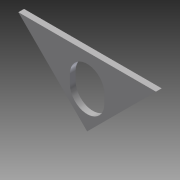
# Autodesk Inventor part: GE-13020-02
Saved by Autodesk Inventor 2013 (Build 170138000, 138)
## iProperties
Created: 2013-01-06
Part Number: GE-13020-02
Material: Steel
Document SubType Name: Modeling
Designer: Phillip
Density: 1 g/cm^3
Author: Phillip
Autodesk Inventor part; units mm, degrees
ref_plane "YZ Plane" through (0, 0, 0) normal (1, 0, 0) x (0, 1, 0)
ref_plane "XZ Plane" through (0, 0, 0) normal (0, 1, 0) x (-1, 0, 0)
ref_plane "XY Plane" through (0, 0, 0) normal (0, 0, 1) x (1, 0, 0)
sketch "Sketch1" plane through (0, 0, 0) normal (0, 0, 1) x (1, 0, 0)
  line L0 (0, 0) -> (-76.2, 76.2)
  line L1 (-76.2, 76.2) -> (76.2, 76.2)
  line L2 (76.2, 76.2) -> (0, 0)
  point P0 (0, 76.2)
  dimension "d0" = 152.4
  dimension "d2" = 76.2
  constraints: 6 end point, 1 horizontal, 1 midpoint, 1 vertical alignment
  measures "d0" distance of L0.end L1.end
  measures "d2" distance from line of L0.start L1
extrude "Extrusion1" add sketch "Sketch1" against normal blind 6.35
sketch "Sketch2" plane through (0, 0, 0) normal (0, 0, 1) x (1, 0, 0)
  line L0 (-76.2, 76.2) -> (76.2, 76.2) projected
  line L1 (-19.05, 35.56) -> (-19.05, 45.72)
  arc A0 (19.05, 45.72) -> (-19.05, 45.72) centre (0, 45.72) ccw
  line L2 (19.05, 45.72) -> (19.05, 35.56)
  arc A1 (-19.05, 35.56) -> (19.05, 35.56) centre (0, 35.56) ccw
  point P0 (0, 76.2)
  dimension "d5" = 10.16
  dimension "d6" = 19.05
  dimension "d7" = 30.48
  constraints: 4 end point, 4 point on circle, 4 tangent, 2 centre point, 1 midpoint, 1 parallel, 1 perpendicular, 1 vertical alignment
  measures "d5" distance of L1.start L1.end
  measures "d6" radius of A0
  measures "d7" distance from line of A0.centre L0
extrude "Extrusion2" cut sketch "Sketch2" against normal through all
ref_plane "Work Plane1" through (76.2, 76.2, -3.175) normal (0, 0, -1) x (-1, 0, 0)
body "Solid1"
